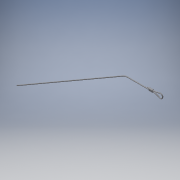
# Autodesk Inventor part: wire
Saved by Autodesk Inventor 2018 (Build 220112000, 112)
## iProperties
Created: 2018-06-15
Part Number: wire
Material: 一般
Document SubType Name: Modeling
Designer: KITformula
Density: 1 g/cm^3
Appearance: 既定
Author: KITformula
Autodesk Inventor part; units mm, degrees
ref_plane "YZ Plane" through (0, 0, 0) normal (1, 0, 0) x (0, 1, 0)
ref_plane "XZ Plane" through (0, 0, 0) normal (0, 1, 0) x (-1, 0, 0)
ref_plane "XY Plane" through (0, 0, 0) normal (0, 0, 1) x (1, 0, 0)
sketch "スケッチ1" plane through (0, 0, 0) normal (1, 0, 0) x (0, 1, 0)
  circle A0 centre (0, 0) radius 1.25
  dimension "d0" = 2.5
  constraints: 1 centre point, 1 coincident
  measures "d0" diameter of A0
extrude "押し出し1" add sketch "スケッチ1" along normal mid plane 100
sketch "スケッチ2" plane through (50, 0, 0) normal (1, 0, 0) x (0, 0, -1)
  circle A0 centre (0, 0) radius 1.25 projected
sketch "スケッチ3" plane through (0, 0, 0) normal (0, 1, 0) x (-1, 0, 0)
  line L0 (-50, 1.25) -> (-50, -1.25) projected
  arc A0 (-50, 0) -> (-66.932, -4.6563) centre (-50, -33.1136) ccw
  arc A1 (-67.9624, 6.1434) -> (-66.932, -4.6563) centre (-70, 0.5) ccw
  arc A2 (-67.9624, 6.1434) -> (-50, 3) centre (-50, 55.8929) ccw
  line L1 (-50, 3) -> (-40, 3)
  point P0 (0, 0)
  dimension "d3" = 3
  dimension "d4" = 20
  dimension "d5" = 2.5
  dimension "d8" = 10
  dimension "d21" = 6
  constraints: 6 point on circle, 3 centre point, 3 tangent, 2 end point, 1 horizontal, 1 line through centre, 1 midpoint, 1 point on line
  measures "d3" distance from line of A0.start L1
  measures "d4" distance from line of A1.centre L0
  measures "d5" distance from line of A1.centre L1
  measures "d8" distance of L1.start L1.end
  measures "d21" radius of A1
sweep "スイープ1" add profiles "スケッチ2" path "スケッチ3" path curves A0 A1 A2 L1
sketch "スケッチ4" plane through (40, 0, 3) normal (-1, 0, 0) x (0, 0, 1)
  line L0 (-5, -2.5) -> (2, -2.5)
  line L1 (2, -2.5) -> (2, 2.5)
  line L2 (2, 2.5) -> (-5, 2.5)
  line L3 (-5, 2.5) -> (-5, -2.5)
  line L4 (-5, -2.5) -> (2, 2.5) construction
  line L5 (2, -2.5) -> (-5, 2.5) construction
  circle A0 centre (0, 0) radius 1.25 projected
  line L6 (-12.65, 0) -> (7.65, 0) projected
  point P0 (-3, 0)
  point P1 (-1.5, 0)
  point P2 (-1.5, 0)
  dimension "d9" = 1.5
  dimension "d10" = 7
  dimension "d11" = 5
  constraints: 12 end point, 3 midpoint, 2 parallel, 1 horizontal, 1 perpendicular, 1 point on line
  measures "d9" distance of A0.centre point (-1.5, 0)
  measures "d10" distance of L1.end L2.end
  measures "d11" distance of L2.end L0.start
extrude "押し出し2" add sketch "スケッチ4" against normal blind 10
fillet "フィレット1" radius 2 4 edges at (45, 2.5, -2) (45, -2.5, -2) (45, -2.5, 5) (45, 2.5, 5)
sketch "スケッチ5" plane through (40, 0, 3) normal (1, 0, 0) x (0, 0, 1)
  circle A0 centre (0, 0) radius 1.25 projected
  point P0 (-3, 0)
extrude "押し出し3" add sketch "スケッチ5" against normal blind 5
sketch "スケッチ6" plane through (0, 0, 0) normal (0, 1, 0) x (-1, 0, 0)
  line L0 (50, -1.25) -> (50, 1.25) projected
  arc A0 (60, -2.6795) -> (50, 0) centre (50, -20) ccw
  line L1 (60, -2.6795) -> (349.5135, -169.8302)
  line L2 (50, 1.25) -> (-40, 1.25) projected
  point P0 (0, 0)
  dimension "d17" = 30
  dimension "d18" = 20
  constraints: 2 end point, 2 point on circle, 1 centre point, 1 line through centre, 1 midpoint, 1 tangent
  measures "d17" angle of L1 L2
  measures "d18" radius of A0
sketch "スケッチ7" plane through (-50, 0, 0) normal (-1, 0, 0) x (0, 0, 1)
  circle A0 centre (0, 0) radius 1.25 projected
sweep "スイープ2" add profiles "スケッチ7" path "スケッチ6" path curves A0 L1
